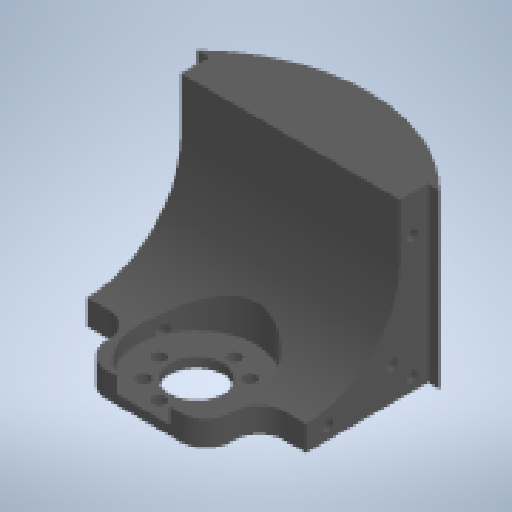
# Autodesk Inventor part: toe_joint_middle
Saved by Autodesk Inventor 2024.1 (Build 281209000, 209)
## iProperties
Created: 2024-02-11
Part Number: toe_joint_middle
Material: 一般
Document SubType Name: Modeling
Designer: hibik
Density: 1 g/cm^3
Appearance: 既定
Author: hibik
Autodesk Inventor part; units mm, degrees
ref_plane "YZ Plane" through (0, 0, 0) normal (1, 0, 0) x (0, 1, 0)
ref_plane "XZ Plane" through (0, 0, 0) normal (0, 1, 0) x (-1, 0, 0)
ref_plane "XY Plane" through (0, 0, 0) normal (0, 0, 1) x (1, 0, 0)
sketch "スケッチ1" plane through (0, 0, 0) normal (0, 1, 0) x (-1, 0, 0)
  line L0 (17.5, 8.5) -> (-17.5, 8.5)
  line L1 (-17.5, 8.5) -> (-17.5, -8.5)
  line L2 (-17.5, -8.5) -> (17.5, -8.5)
  line L3 (17.5, -8.5) -> (17.5, 8.5)
  line L4 (17.5, 8.5) -> (-17.5, -8.5) construction
  line L5 (-17.5, 8.5) -> (17.5, -8.5) construction
  point P0 (0, 0)
  dimension "d0" = 17
  dimension "d1" = 35
  constraints: 12 end point, 2 midpoint, 2 parallel, 1 horizontal, 1 perpendicular
  measures "d0" distance of L2.end L0.start
  measures "d1" distance of L1.end L2.end
extrude "押し出し1" add sketch "スケッチ1" along normal blind 4
sketch "スケッチ3" plane through (-17.5, 0, -8.5) normal (-1, 0, 0) x (0, 0, 1)
  line L0 (17, 19) -> (0, 19)
  line L1 (0, 19) -> (0, 0)
  line L2 (0, 0) -> (17, 0)
  line L3 (17, 0) -> (17, 19)
  line L4 (0, 0) -> (17, 0) projected
  line L5 (17, 0) -> (17, 4) projected
  line L6 (0, 4) -> (17, 4) projected
  circle A0 centre (8.5, 19) radius 15
  line L7 (-6.5, 27.5) -> (-21.5, 27.5)
  line L8 (-21.5, 27.5) -> (-21.5, 0)
  line L9 (-21.5, 0) -> (-6.5, 0)
  line L10 (-6.5, 0) -> (-6.5, 27.5)
  line L11 (0, 4) -> (-6.5, 4)
  line L12 (-6.5, 4) -> (-6.5, 0)
  line L13 (-6.5, 0) -> (0, 0)
  line L14 (0, 0) -> (0, 4)
  line L15 (0, 0) -> (0, 4) projected
  point P0 (8.5, 0)
  dimension "d4" = 15
  dimension "d5" = 30
  dimension "d6" = 15
  dimension "d7" = 27.5
  constraints: 24 end point, 6 parallel, 4 collinear, 3 horizontal, 3 perpendicular, 1 centre point, 1 midpoint, 1 point on line, 1 tangent
  measures "d4" distance between parallel lines of L6 L0
  measures "d5" diameter of A0
  measures "d6" distance of L7.start L7.end
  measures "d7" distance of L7.end L8.end
extrude "押し出し2" add sketch "スケッチ3" against normal blind 35 contours L1 L13 L10 L11 | L10 L9 L8 L7
sketch "スケッチ5" plane through (0, 0, 0) normal (0, -1, 0) x (1, 0, 0)
  circle A0 centre (0, 0) radius 4.25
  circle A1 centre (0, 0) radius 6
  circle A2 centre (0, 6) radius 1
  line L0 (0, -41.5) -> (0, 39) projected
  circle A3 centre (-4.2426, 4.2426) radius 1
  circle A4 centre (-6, 0) radius 1
  circle A5 centre (-4.2426, -4.2426) radius 1
  circle A6 centre (0, -6) radius 1
  circle A7 centre (4.2426, -4.2426) radius 1
  circle A8 centre (0, 0) radius 23.0489
  circle A9 centre (0, 0) radius 27.5
  line L1 (-17.5, -30) -> (-17.5, 8.5) projected
  line L2 (17.5, 8.5) -> (17.5, -30) projected
  line L3 (-17.5, 8.5) -> (17.5, 8.5) projected
  line L4 (-17.5, -30) -> (-17.5, 8.5) projected
  line L5 (-17.5, -30) -> (17.5, -30) projected
  line L6 (17.5, 8.5) -> (17.5, -15) projected
  line L7 (17.5, 8.5) -> (19.3907, 8.5)
  line L8 (19.3907, 8.5) -> (19.3907, -19.5)
  line L9 (19.3907, -19.5) -> (17.5, -19.5)
  line L10 (17.5, -19.5) -> (17.5, 8.5)
  line L11 (-17.5, 8.5) -> (-19.3907, 8.5)
  line L12 (-19.3907, 8.5) -> (-19.3907, -19.5)
  line L13 (-19.3907, -19.5) -> (-17.5, -19.5)
  line L14 (-17.5, -19.5) -> (-17.5, 8.5)
  circle A10 centre (6, 0) radius 1
  circle A11 centre (4.2426, 4.2426) radius 1
  point P0 (17.5, -21.2132)
  point P1 (-17.5, -21.2132)
  dimension "d11" = 12
  dimension "d18" = 46.0977
  dimension "d10" = 8.5
  dimension "d12" = 2
  dimension "d15" = 360
  dimension "d17" = 55
  dimension "d36" = 4.5
  constraints: 16 end point, 10 centre point, 4 coincident, 4 parallel, 3 point on line, 2 horizontal, 2 perpendicular, 2 point on circle, 1 vertical alignment, 23 other
  measures "d10" diameter of A0
  measures "d12" diameter of A2
  measures "d17" diameter of A9
  measures "d36" vertical distance of L8.end L6.end
extrude "押し出し3" cut sketch "スケッチ5" against normal through all contours A0 L0 | L0 A0 | L0 A1 A2 | A2 A1 L0 | A6 A1 L0 | L0 A1 A6 | A2 L0 A1 | A1 L0 A2 | L0 A6 A1 | A1 A6 L0 | A3 A1 | A1 A3 | A11 A1 | A1 A11 | A7 A1 | A1 A7 | A5 A1 | A1 A5 | A4 A1 | A1 A4 | A10 A1 | A1 A10 | A9 L2 L5 L0 | L0 L5 L1 A9
extrude "押し出し6" add sketch "スケッチ5" against normal up to surface (27.5 mm away) contours A9 L13 L1 | L2 L9 A9
sketch "スケッチ6" plane through (0, 4, 0) normal (0, 1, 0) x (1, 0, 0)
  circle A0 centre (0, 0) radius 9.5
  dimension "d21" = 19
  constraints: 1 centre point, 1 coincident
  measures "d21" diameter of A0
extrude "押し出し4" cut sketch "スケッチ6" against normal blind 2.5
sketch "スケッチ7" plane through (0, 0, 0) normal (0, -1, 0) x (1, 0, 0)
  line L0 (-10, 8.5) -> (10, 8.5)
  line L1 (10, 8.5) -> (10, 0)
  line L2 (10, 0) -> (-10, 0)
  line L3 (-10, 0) -> (-10, 8.5)
  line L4 (0, -27.1558) -> (0, 14.4426) projected
  line L5 (-17.5, 8.5) -> (17.5, 8.5) projected
  line L6 (17.5, 8.5) -> (17.5, -21.2132) projected
  line L7 (10, 8.5) -> (17.5, 8.5)
  line L8 (17.5, 8.5) -> (17.5, 0)
  line L9 (17.5, 0) -> (10, 0)
  line L10 (10, 0) -> (10, 8.5)
  line L11 (-17.5, 8.5) -> (-17.5, -15) projected
  line L12 (-10, 8.5) -> (-17.5, 8.5)
  line L13 (-17.5, 8.5) -> (-17.5, 0)
  line L14 (-17.5, 0) -> (-10, 0)
  line L15 (-10, 0) -> (-10, 8.5)
  point P0 (0, 0)
  point P1 (0, 8.5)
  point P2 (-17.5, -12)
  point P3 (10, 8.5)
  point P4 (-10, 8.5)
  dimension "d27" = 20
  constraints: 24 end point, 6 parallel, 4 point on line, 3 horizontal, 3 perpendicular, 2 collinear, 2 midpoint
  measures "d27" distance of L0.start L0.end
extrude "押し出し5" cut sketch "スケッチ7" against normal through all contours L3 L14 L11 L5 | L5 L6 L9 L1
fillet "フィレット1" radius 4 4 edges at (10, 2, 0) (10, 2, 8.5) (-10, 2, 8.5) (-10, 2, 0)
fillet "フィレット2" radius 15 1 edges at (0, 4, -15)
sketch "スケッチ8" plane through (17.5, 0, -19.5) normal (1, 0, 0) x (0, 0, -1)
  circle A0 centre (-16, 2) radius 0.8
  circle A1 centre (-2.5, 2) radius 0.8
  circle A2 centre (-2.5, 21.5) radius 0.8
  line L0 (-4.5, 27.5) -> (-4.5, 19) projected
  line L1 (-19.5, 4) -> (-23.5, 4) projected
  line L2 (0, 27.5) -> (-4.5, 27.5) projected
  line L3 (-28, 4) -> (-28, 0) projected
  circle A3 centre (-5.6967, 5.1967) radius 0.8
  arc A4 (-4.566, 17.5947) -> (-4.6176, 20.875) centre (-19.5, 19) ccw projected
  line L4 (-19.5, 19) -> (-2.5, 2)
  arc A5 (-19.5, 4) -> (-4.5, 19) centre (-19.5, 19) ccw projected
  point P0 (-19.5, 0)
  point P1 (-8.8934, 8.3934)
  dimension "d39" = 1.6
  dimension "d40" = 1.6
  dimension "d41" = 1.6
  dimension "d42" = 2
  dimension "d43" = 2
  dimension "d44" = 6
  dimension "d45" = 12
  dimension "d46" = 1.6
  dimension "d48" = 13.8033
  dimension "d49" = 17
  dimension "d50" = 10.6066
  constraints: 4 centre point, 2 end point, 1 horizontal alignment, 1 point on circle, 1 point on line, 1 vertical alignment
  measures "d39" diameter of A0
  measures "d40" diameter of A1
  measures "d41" diameter of A2
  measures "d42" distance from line of L0 A2.centre
  measures "d43" distance from line of L1 A0.centre
  measures "d44" distance from line of L2 A2.centre
  measures "d45" distance from line of L3 A0.centre
  measures "d46" diameter of A3
  measures "d48" horizontal distance of L4.start A3.centre
  measures "d49" horizontal distance of L4.start L4.end
  measures "d50" horizontal distance of L4.start point (-8.893, 8.393)
extrude "押し出し7" cut sketch "スケッチ8" against normal through all
sketch "スケッチ9" plane through (0, 1.5, 0) normal (0, 1, 0) x (1, 0, 0)
  spline S0 degree 6 poles (9.5, 0) (9.5, 0.6679) (9.4437, 1.3293) (9.333, 1.9745) (9.1731, 2.5937) (8.972, 3.1782) (8.5497, 4.1702) (8.3362, 4.5949) (8.104, 4.9949) (7.8558, 5.371) (7.5939, 5.7242) (6.9979, 6.4447) (6.6588, 6.8041) (6.305, 7.1351) (5.9383, 7.4391) (5.5596, 7.7174) (4.7818, 8.2218) (4.3828, 8.4484) (3.9735, 8.6506) (3.5549, 8.8284) (3.1279, 8.9818) (2.2576, 9.239) (1.8142, 9.3429) (1.3649, 9.4213) (0.9116, 9.4737) (0.456, 9.5) (-0.45, 9.5) (-0.8994, 9.4744) (-1.3468, 9.4234) (-1.7903, 9.3471) (-2.2281, 9.2459) (-3.0994, 8.9919) (-3.5326, 8.8379) (-3.9572, 8.6587) (-4.3722, 8.4545) (-4.7767, 8.2251) (-5.6955, 7.6292) (-6.2002, 7.2426) (-6.6829, 6.8088) (-7.1409, 6.3243) (-7.5691, 5.7851) (-8.2204, 4.7858) (-8.4657, 4.3564) (-8.6907, 3.8989) (-8.8913, 3.4137) (-9.0632, 2.9012) (-9.2971, 1.9902) (-9.3767, 1.6055) (-9.4378, 1.2111) (-9.4792, 0.8101) (-9.5, 0.4054) (-9.5, 0) knots 0 0 0 0 0 0 0 0.105424 0.105424 0.105424 0.105424 0.105424 0.1929 0.1929 0.1929 0.1929 0.1929 0.295669 0.295669 0.295669 0.295669 0.295669 0.397708 0.397708 0.397708 0.397708 0.397708 0.499807 0.499807 0.499807 0.499807 0.499807 0.600545 0.600545 0.600545 0.600545 0.600545 0.70394 0.70394 0.70394 0.70394 0.70394 0.842489 0.842489 0.842489 0.842489 0.842489 0.935619 0.935619 0.935619 0.935619 0.935619 1 1 1 1 1 1 1 projected
  arc A0 (-9.5, 0) -> (-4.2426, -8.5) centre (0, 0) ccw projected
  arc A1 (4.2426, -8.5) -> (9.5, 0) centre (0, 0) ccw projected
  line L0 (4.2426, -8.5) -> (-4.2426, -8.5) projected
  arc A2 (8.5579, 4.1245) -> (-8.5579, 4.1245) centre (0, 0) ccw projected
  arc A3 (4.2426, -8.5) -> (9.0544, 2.8755) centre (0, 0) ccw projected
  arc A4 (-3.2496, 4.1245) -> (-5.2356, 4.1245) centre (-4.2426, 4.2426) ccw projected
  circle A5 centre (0, 6) radius 1 projected
  circle A6 centre (4.2426, 4.2426) radius 1 projected
  circle A7 centre (0, -6) radius 1 projected
  circle A8 centre (-4.2426, -4.2426) radius 1 projected
  circle A9 centre (-6, 0) radius 1 projected
  circle A10 centre (0, 0) radius 4.25 projected
  circle A11 centre (0, 0) radius 9.5
  spline S1 degree 5 poles (-5.2356, 4.1245) (-5.2254, 4.0383) (-5.2033, 3.9297) (-5.1576, 3.8033) (-5.0832, 3.6824) (-4.8791, 3.4542) (-4.7425, 3.352) (-4.5863, 3.2799) (-4.4144, 3.2426) (-4.0708, 3.2426) (-3.899, 3.2799) (-3.7428, 3.352) (-3.6062, 3.4542) (-3.4021, 3.6824) (-3.3277, 3.8033) (-3.282, 3.9297) (-3.2599, 4.0383) (-3.2496, 4.1245) knots 0 0 0 0 0 0 0.233643 0.233643 0.233643 0.233643 0.5 0.5 0.5 0.5 0.766357 0.766357 0.766357 0.766357 1 1 1 1 1 1 projected
  circle A12 centre (6, 0) radius 1 projected
  circle A13 centre (4.2426, -4.2426) radius 1 projected
  point P0 (9.0544, 2.8755)
  point P1 (8.5579, 4.1245)
  point P2 (-0.7994, 9.4663)
  point P3 (0, 9.5)
  constraints: 6 coincident, 1 centre point, 1 concentric, 1 horizontal alignment, 1 other
extrude "押し出し8" add sketch "スケッチ9" against normal up to surface (1.5 mm away) contours A1 L0 A0 S0
equation "\"d48\" = 0.5 * d50 + 0.5 * d49"
